Semana2_DesafioExtra (Autodesk Fusion 360 design; units mm, degrees)
Autodesk Fusion 360 part; units mm, degrees
sketch "Sketch1" plane through (0, 0, 0) normal (0, 0, 1) x (1, 0, 0)
  line L0 (0, 14) -> (0, -14) construction
  spline S0 degree 5 poles (0, -11) (0.2848, -10.9655) (0.8331, -10.8977) (1.5913, -10.7995) (2.4774, -10.6745) (3.3963, -10.5201) (4.1534, -10.3574) (4.7787, -10.1766) (5.3012, -9.9695) (5.7436, -9.7338) (6.121, -9.4705) (6.429, -9.1983) (6.6607, -8.9222) (6.8298, -8.6073) (6.9572, -8.2126) (7.0699, -7.7028) (7.1951, -7.0718) (7.3509, -6.3188) (7.5471, -5.4539) (7.7842, -4.4976) (8.0513, -3.4826) (8.3282, -2.4546) (8.5784, -1.4738) (8.7611, -0.6153) (8.8008, 0.0282) (8.6558, 0.347) (8.4721, 0.3481) (8.3493, 0.2228) (8.1811, 0.4712) (8.0648, 0.8572) (8.0614, 1.0698) (7.8242, 1.5037) (7.4182, 2.0123) (7.0567, 2.326) (6.9707, 2.2142) (7.0198, 2.2474) (7.0907, 2.6767) (7.1861, 3.2501) (7.279, 3.6826) (7.0687, 4.13) (6.5468, 4.6109) (5.9466, 4.963) (5.5113, 5.0915) (5.4092, 4.9933) (5.4203, 5.1198) (5.3971, 5.5868) (5.2904, 6.2398) (5.0741, 6.8556) (4.7054, 7.2803) (4.0876, 7.603) (3.3779, 7.8066) (2.7924, 7.879) (2.4993, 7.8479) (2.5291, 7.8042) (2.5431, 8.0376) (2.3937, 8.5144) (2.0681, 9.0572) (1.6303, 9.4625) (1.1701, 9.7049) (0.7472, 9.938) (0.3974, 10.207) (0.1902, 10.4827) (0.0782, 10.7266) (0.0228, 10.9061) (0, 11) knots 0 0 0 0 0 0 0.01666667 0.03333333 0.05 0.06666667 0.08333333 0.1 0.11666667 0.13333333 0.15 0.16666667 0.18333333 0.2 0.21666667 0.23333333 0.25 0.26666667 0.28333333 0.3 0.31666667 0.33333333 0.35 0.36666667 0.38333333 0.4 0.41666667 0.43333333 0.45 0.46666667 0.48333333 0.5 0.51666667 0.53333333 0.55 0.56666667 0.58333333 0.6 0.61666667 0.63333333 0.65 0.66666667 0.68333333 0.7 0.71666667 0.73333333 0.75 0.76666667 0.78333333 0.8 0.81666667 0.83333333 0.85 0.86666667 0.88333333 0.9 0.91666667 0.93333333 0.95 0.96666667 0.98333333 1 1 1 1 1 1
  line L1 (-4.8078, -11.5824) -> (4.8078, -10.4176)
  line L2 (6.5595, -9.8482) -> (7.4405, -6.1518)
  line L3 (4.7855, -10.509) -> (7.4576, -8.3992)
  line L4 (9.5, 0.5) -> (7.33, 0.1027)
  line L5 (8.6662, -1.3172) -> (7.4336, 3.2939)
  line L6 (8.5, -3) -> (8.9984, 2.0471)
  line L7 (7.28, 2.3213) -> (6.7432, 2.1779)
  line L8 (7.2417, 0.9004) -> (7.1911, 6.2047)
  line L9 (5.9939, 5.0415) -> (4.9354, 5.0415)
  line L10 (6.9063, 4.5) -> (2.9063, 9.5)
  line L11 (2.6868, 7.6899) -> (2.3743, 7.9988)
  line L12 (4.2372, 7.5919) -> (-1.1031, 11.3374)
  line L13 (0, 11) -> (0, -11)
  point P0 (0, 11)
  point P1 (1.5671, 9.4647)
  point P2 (2.5305, 7.8443)
  point P3 (5.4647, 5.0415)
  point P4 (8.7607, -0.1093)
  point P5 (8.7607, -0.4764)
  point P6 (7, -8)
  point P7 (6.1216, -9.4541)
  point P8 (0, -11)
  point P9 (6.1216, -9.4541)
  point P10 (7, -8)
  point P11 (8.7492, -0.4764)
  point P12 (8.415, 0.3014)
  point P13 (8.0499, 0.9883)
  point P14 (7.0116, 2.2496)
  point P15 (7.2164, 3.5526)
  point P16 (5.4647, 5.0415)
  point P17 (4.9063, 7)
  point P18 (2.5305, 7.8443)
  point P19 (1.5671, 9.4647)
  constraint vertical L0
  constraint coincident L0 P0
  constraint vertical P4 P5
  constraint coincident L0 P8
  constraint coincident P19 P1
  constraint coincident P0 S0.end
  constraint midpoint P8 L1
  constraint midpoint P10 L2
  constraint midpoint P9 L3
  constraint midpoint P12 L4
  constraint coincident P4 S0
  constraint midpoint P13 L5
  constraint midpoint P11 L6
  constraint coincident L5.start L6
  constraint midpoint P14 L7
  constraint midpoint P15 L8
  constraint midpoint P16 L9
  constraint perpendicular L5 L7
  constraint midpoint P17 L10
  constraint midpoint P18 L11
  constraint midpoint P19 L12
  constraint coincident P8 S0.start
revolve "Revolve1" add sketch "Sketch1" angle 360 about axis through (0, 14, 0) along (0, -1, 0) contours S0 L5 L12 L13 | S0 L12 L13 | S0 L4 L5 | S0 L4 L5 | S0 L4
